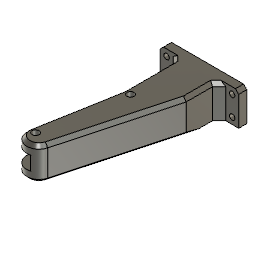
GRIP ARM (Autodesk Fusion 360 design; units mm, degrees)
part number: 2026-03-21-14-20-57-704
Autodesk Fusion 360 part; units mm, degrees
note: some values were not read from the file. Set by a fixed rule: which sketch regions a step uses.
sketch "Sketch1" plane through (0, 0, 0) normal (0, 0, 1) x (1, 0, 0)
  line L0 (-17, 40) -> (-17, 35)
  line L1 (-5, 0) -> (-13.6051, -48.3645)
  line L2 (-5, 35) -> (-17, 35)
  line L3 (-6.5651, -49.6137) -> (-6.2204, -49.6745)
  circle A0 centre (0, 0) radius 2.15
  line L4 (23, 35) -> (19, 35)
  circle A1 centre (-8.6824, -49.2404) radius 2.15
  line L5 (19, 15) -> (1.0206, -51.6285)
  line L6 (9.1345, 0) -> (2.15, 0)
  line L7 (31, 40) -> (-17, 40)
  line L8 (19, 35) -> (19, 15)
  line L9 (31, 35) -> (31, 40)
  line L10 (5, 35) -> (-5, 35)
  line L11 (31, 35) -> (19, 35)
  line L12 (-5, 35) -> (-5, 0)
  arc A2 (-13.6051, -48.3645) -> (-13.6064, -48.3721) centre (-8.6824, -49.2404) ccw
  arc A3 (-13.6044, -48.3607) -> (1.0206, -51.6285) centre (-6.2204, -49.6745) ccw
  line L13 (-5, 0) -> (-2.15, 0)
  line L14 (2.15, 0) -> (5, 0)
  line L15 (-17, 35) -> (-5, 35)
  line L16 (19, 35) -> (31, 35)
  line L17 (-17, 35) -> (-5, 35)
  line L18 (19, 35) -> (31, 35)
  dimension "d1" = 4.3
  dimension "d2" = 48
  dimension "d4" = 5
  dimension "d5" = 4.3
  dimension "d6" = 10
  dimension "d7" = 12
  dimension "d9" = 50
  dimension "d10" = 15
  dimension "d11" = 20
  constraint coincident A0.centre origin
  constraint horizontal L15
  constraint vertical L9
  constraint horizontal L7
  constraint vertical L0
  constraint coincident L9.start L11.start
  constraint horizontal L13
  constraint horizontal L10
  constraint vertical L12
  constraint coincident L10.start L17
  constraint horizontal L4
  constraint coincident L4.start L16
  constraint concentric A1 A2
  constraint tangent L1 A2
  constraint perpendicular L9 L11
  constraint perpendicular L4 L8
  constraint tangent L5 A3
  constraint coincident L3.end A3.centre
  constraint tangent L1 A3
  constraint equal L2 L11
  constraint coincident A2.end A3
  constraint coincident L1 A3.start
  constraint coincident A0 L6.end
  constraint coincident A0 L13.end
  constraint collinear L13 L14
  constraint collinear L15 L16
  constraint collinear L17 L18
  constraint coincident A1 L3.start
  measures "d1" diameter of A0
  measures "d2" distance of L9.start L0.end
  measures "d4" distance of L7.start L9.start
  measures "d5" diameter of A1
  measures "d6" diameter of A2
  measures "d7" distance of L4.end L9.start
  measures "d9" distance of A1.centre A0.centre
  measures "d10" diameter of A3
  measures "d11" distance of L5.start L4.end
extrude "Extrude1" add sketch "Sketch1" along normal mid plane 20
sketch "Sketch2" plane through (0, 40, 0) normal (0, 1, 0) x (-1, 0, 0)
  line L0 (17, -10) -> (17, 10)
  line L1 (17, 10) -> (-31, 10)
  line L2 (-31, 10) -> (-31, -10)
  line L3 (-31, -10) -> (17, -10)
  circle A0 centre (-27, -6) radius 1.65
  circle A1 centre (13, 6) radius 1.65
  line L4 (13, 6) -> (13, -6)
  line L5 (-7, 0) -> (-7, -6)
  line L6 (-7, 0) -> (-31, 0)
  line L7 (13, -6) -> (-27, -6)
  line L8 (-27, 6) -> (13, 6)
  line L9 (-7, 0) -> (-7, -10)
  line L10 (-31, -10) -> (17, -10)
  line L11 (-31, 10) -> (-31, -10)
  line L12 (-7, 0) -> (-27, 0)
  line L13 (17, -10) -> (17, 10)
  line L14 (17, 10) -> (-31, 10)
  circle A2 centre (13, -6) radius 1.65
  circle A3 centre (-27, 6) radius 1.65
  line L15 (-27, -6) -> (-27, 6)
  dimension "d15" = 40
  dimension "d16" = 12
  dimension "d17" = 3.3
  dimension "d18" = 3.3
  dimension "d19" = 3.3
  dimension "d20" = 3.3
  constraint perpendicular L9 L10
  constraint perpendicular L6 L9
  constraint midpoint L9.end L10
  constraint midpoint L6.end L11
  constraint horizontal L7
  constraint vertical L15
  constraint horizontal L8
  constraint vertical L4
  constraint coincident L5.end L9
  constraint coincident L12.end L6
  constraint midpoint L5.end L7
  constraint midpoint L12.end L15
  constraint coincident A0.centre L7.end
  constraint coincident L4.end L7.start
  constraint coincident A1.centre L4.start
  constraint coincident L8.start A3.centre
  measures "d15" distance of A0.centre L4.end
  measures "d16" distance of L8.start A0.centre
  measures "d17" diameter of A0
  measures "d18" diameter of A2
  measures "d19" diameter of A1
  measures "d20" diameter of A3
extrude "Extrude2" cut sketch "Sketch2" against normal up to surface (5 mm away) contours A0 L7 L15 | A0 L7 L15 | L4 L7 A2 | L4 L7 A2 | L8 A3 L15 | L8 A3 L15 | A1 L4 L8 | A1 L4 L8
chamfer "Chamfer1" distance 4 angle 45 2 edges at (-5, 35, 0) (19, 35, 0)
chamfer "Chamfer2" distance 2 angle 45 15 edges at (-7, 33, -10) (-17, 37.5, -10) (-5, 15.5, -10) (-9.3022, -24.1804, -10) (10.0103, -18.3142, -10) (-7.8558, -56.994, -10) (-5, 15.5, 10) (-9.3022, -24.1804, 10) (-7.8558, -56.994, 10) (10.0103, -18.3142, 10) (-7, 33, 10) (-17, 37.5, 10) (31, 37.5, 10) (21, 33, 10) (19, 23, 10)
sketch "Sketch3" plane through (0, 0, 0) normal (0, 0, 1) x (1, 0, 0)
  line L0 (-14, -82) -> (-2.1648, -51.7941)
  circle A0 centre (-8.6824, -49.2404) radius 7
  line L1 (-14, -82) -> (-60, -70)
  line L2 (9, 21) -> (6.9694, -0.6536)
  line L3 (-60, -70) -> (-51.4576, 32.3922)
  line L4 (-18, 34) -> (9, 21)
  line L5 (-9.4078, -10.4426) -> (2.1764, -6.6531)
  line L6 (-51.4576, 32.3922) -> (-18, 34)
  circle A1 centre (0, 0) radius 7
  line L7 (-10, -14) -> (-1.8784, -47.5955)
  line L8 (-9.4078, -10.4426) -> (-10, -14)
  circle A2 centre (0, 0) radius 2.15
  circle A3 centre (-8.6824, -49.2404) radius 2.15
  dimension "d25" = 14
  dimension "d26" = 14
  constraint coincident L2.end A1
  constraint tangent L2 A1
  constraint coincident L5.end A1
  constraint tangent L5 A1
  constraint coincident L7.end A0
  constraint tangent A0 L7
  constraint coincident L0.end A0
  constraint tangent L0 A0
  constraint coincident A1.centre A2.centre
  measures "d25" diameter of A0
  measures "d26" diameter of A1
extrude "Extrude3" cut sketch "Sketch3" along normal mid plane 8.5
